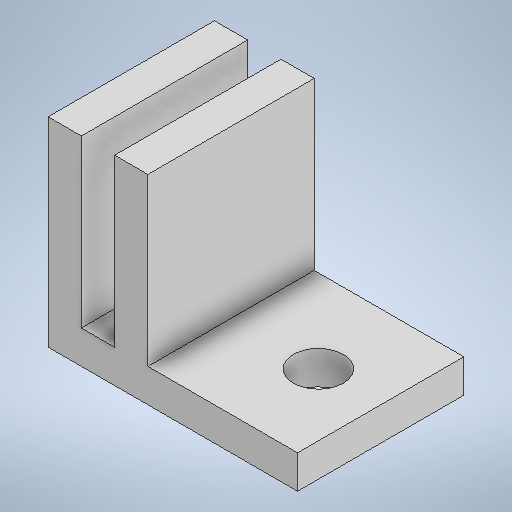
# Autodesk Inventor part: TOF_holder
Saved by Autodesk Inventor 2025 (Build 290162000, 162)
## iProperties
Created: 2026-03-16
Part Number: TOF_holder
Material: Générique
Document SubType Name: Modeling
Designer: luc4s
Density: 1 g/cm^3
Appearance: Par défaut
Author: luc4s
Autodesk Inventor part; units mm, degrees
ref_plane "YZ Plane" through (0, 0, 0) normal (1, 0, 0) x (0, 1, 0)
ref_plane "XZ Plane" through (0, 0, 0) normal (0, 1, 0) x (-1, 0, 0)
ref_plane "XY Plane" through (0, 0, 0) normal (0, 0, 1) x (1, 0, 0)
sketch "Esquisse1" plane through (0, 0, 0) normal (0, 1, 0) x (-1, 0, 0)
  line L0 (7.5, 5) -> (-7.5, 5)
  line L1 (-7.5, 5) -> (-7.5, -5)
  line L2 (-7.5, -5) -> (7.5, -5)
  line L3 (7.5, -5) -> (7.5, 5)
  line L4 (7.5, 5) -> (-7.5, -5) construction
  line L5 (7.5, -5) -> (-7.5, 5) construction
  point P0 (0, 0)
  point P1 (0, 0)
  dimension "d0" = 10
  dimension "d1" = 15
  constraints: 12 end point, 2 parallel, 1 coincident, 1 horizontal, 1 midpoint, 1 perpendicular
  measures "d0" distance of L2.end L0.start
  measures "d1" distance of L1.end L2.end
extrude "Extrusion1" add sketch "Esquisse1" along normal blind 2
sketch "Esquisse2" plane through (0, 2, 0) normal (0, 1, 0) x (1, 0, 0)
  line L0 (-7.5, 5) -> (-7.5, -5) projected
  line L1 (7.5, 5) -> (-7.5, 5) projected
  line L2 (-7.5, -5) -> (-5.5, -5)
  line L3 (-5.5, -5) -> (-5.5, 5)
  line L4 (-5.5, 5) -> (-7.5, 5)
  line L5 (-7.5, 5) -> (-7.5, -5)
  line L6 (-7.5, -5) -> (7.5, -5) projected
  line L7 (-3.5, -5) -> (-1.5, -5)
  line L8 (-1.5, -5) -> (-1.5, 5)
  line L9 (-1.5, 5) -> (-3.5, 5)
  line L10 (-3.5, 5) -> (-3.5, -5)
  point P0 (0, 0)
  point P1 (-3.5, 5)
  dimension "d4" = 2
  dimension "d5" = 2
  dimension "d6" = 2
  constraints: 16 end point, 4 parallel, 3 point on line, 2 horizontal, 2 perpendicular
  measures "d4" distance between parallel lines of L0 L3
  measures "d5" distance between parallel lines of L8 L10
  measures "d6" distance between parallel lines of L3 L10
extrude "Extrusion2" add sketch "Esquisse2" along normal blind 10 contours L1 L3 L2 L0 | L1 L8 L6 L10
sketch "Esquisse3" plane through (0, 2, 0) normal (0, 1, 0) x (1, 0, 0)
  circle A0 centre (3.75, 0) radius 1.5
  line L0 (-1.5, -5) -> (7.5, -5) projected
  line L1 (7.5, 5) -> (-1.5, 5) projected
  line L2 (0, -5) -> (7.5, 5) construction
  line L3 (7.5, -5) -> (7.5, 5) projected
  line L4 (0, 5) -> (7.5, -5) construction
  point P0 (0, 0)
  point P1 (3.75, 0)
  dimension "d9" = 3
  constraints: 4 end point, 2 point on line, 1 centre point, 1 coincident, 1 midpoint
  measures "d9" diameter of A0
extrude "Extrusion3" cut sketch "Esquisse3" against normal blind 10
